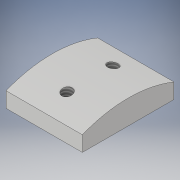
# Autodesk Inventor part: TensionerPusher3
Saved by Autodesk Inventor 2017 (Build 210142000, 142)
## iProperties
Created: 2018-04-06
Part Number: TensionerPusher3
Material: Generic
Document SubType Name: Modeling
Designer: User
Density: 1 g/cm^3
Appearance: Default
Author: User
Autodesk Inventor part; units mm, degrees
ref_plane "YZ Plane" through (0, 0, 0) normal (1, 0, 0) x (0, 1, 0)
ref_plane "XZ Plane" through (0, 0, 0) normal (0, 1, 0) x (-1, 0, 0)
ref_plane "XY Plane" through (0, 0, 0) normal (0, 0, 1) x (1, 0, 0)
sketch "Sketch1" plane through (0, 0, 0) normal (1, 0, 0) x (0, 1, 0)
  line L0 (0, 0) -> (-3.175, 0)
  line L1 (-3.175, 0) -> (-3.175, -19.05)
  line L2 (-3.175, -19.05) -> (0, -19.05)
  arc A0 (0, -19.05) -> (0, 0) centre (-23.5464, -9.525) ccw
  dimension "d4" = 3.175
  dimension "d6" = 25.4
  dimension "d7" = 19.05
  dimension "d23" = 3.175
  constraints: 6 end point, 2 point on circle, 1 centre point, 1 horizontal, 1 parallel, 1 perpendicular
  measures "d4" distance of L2.end L1.end
  measures "d6" radius of A0
  measures "d7" distance of L0.end L1.end
  measures "d23" distance of L0.start L0.end
extrude "Extrusion1" add sketch "Sketch1" along normal blind 15.875
sketch "Sketch2" plane through (0, -3.175, -19.05) normal (0, -1, 0) x (1, 0, 0)
  line L0 (0, 19.05) -> (0, 0) projected
  line L1 (0, 0) -> (15.875, 0) projected
  line L2 (15.875, 19.05) -> (15.875, 0) projected
  line L3 (0, 19.05) -> (15.875, 19.05) projected
  point P0 (7.9375, 14.2875)
  point P1 (7.9375, 4.7625)
  dimension "d10" = 15.875
  dimension "d11" = 7.9375
  dimension "d12" = 7.9375
  dimension "d13" = 9.525
  dimension "d14" = 19.05
  dimension "d15" = 4.7625
  measures "d10" distance of L0.start L2.start
  measures "d11" distance from line of L2 point (7.938, 14.287)
  measures "d12" distance from line of L2 point (7.937, 4.762)
  measures "d13" distance of point (7.937, 4.762) point (7.938, 14.287)
  measures "d14" distance of L2.start L1.end
  measures "d15" distance from line of L3 point (7.938, 14.287)
hole "Hole1" at (7.9375, -3.175, -4.7625) at (7.9375, -3.175, -14.2875) direction (0, 1, 0) diameter 2.159 depth 6.35 tip angle 118
equation "\"d23\" = d4"
equation "\"d11\" = 0.5 * d10"
equation "\"d12\" = d11"
equation "\"d15\" = -0.5 * d13 + 0.5 * d14"
body "Solid1"
